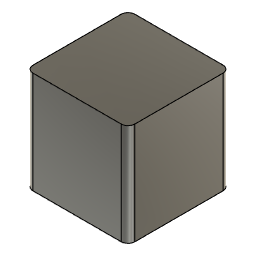
Head v1 (Autodesk Fusion 360 design; units mm, degrees)
Autodesk Fusion 360 part; units mm, degrees
sketch "Sketch1" plane through (0, 0, 0) normal (0, 0, 1) x (1, 0, 0)
  line L0 (15, -15) -> (-15, -15)
  line L1 (-15, -15) -> (-15, 15)
  line L2 (-15, 15) -> (15, 15)
  line L3 (15, 15) -> (15, -15)
  line L4 (15, -15) -> (-15, 15) construction
  line L5 (-15, -15) -> (15, 15) construction
  dimension "d1" = 30
  dimension "d2" = 30
  constraint horizontal L0
  constraint perpendicular L0 L1
  constraint parallel L0 L2
  constraint parallel L1 L3
  constraint coincident L4 origin
  constraint coincident L5 origin
  measures "d1" distance of L1.end L2.end
  measures "d2" distance of L0.end L1.end
extrude "Extrude1" add sketch "Sketch1" along normal blind 30
fillet "Fillet1" radius 2 4 edges at (-15, -15, 15) (15, -15, 15) (15, 15, 15) (-15, 15, 15)
shell "Shell1" thickness 1.6 removed faces 1 at (4.3333, -5, 30)
sketch "Sketch2" plane through (0, 0, 30) normal (0, 0, 1) x (-1, 0, 0)
  arc A0 (-13.4, -13) -> (-13, -13.4) centre (-13, -13) ccw
  line L0 (-13.4, -13) -> (-13.4, 13)
  arc A1 (-13, 13.4) -> (-13.4, 13) centre (-13, 13) ccw
  line L1 (-13, 13.4) -> (13, 13.4)
  arc A2 (13.4, 13) -> (13, 13.4) centre (13, 13) ccw
  line L2 (13.4, 13) -> (13.4, -13)
  arc A3 (13, -13.4) -> (13.4, -13) centre (13, -13) ccw
  line L3 (13, -13.4) -> (-13, -13.4)
  arc A4 (13, -15) -> (15, -13) centre (13, -13) ccw
  line L4 (15, -13) -> (15, 13)
  arc A5 (15, 13) -> (13, 15) centre (13, 13) ccw
  line L5 (13, 15) -> (-13, 15)
  arc A6 (-13, 15) -> (-15, 13) centre (-13, 13) ccw
  line L6 (-15, 13) -> (-15, -13)
  arc A7 (-15, -13) -> (-13, -15) centre (-13, -13) ccw
  line L7 (-13, -15) -> (13, -15)
extrude "Extrude2" add sketch "Sketch2" against normal blind 1.6 contours A0 L0 A1 L1 A2 L2 A3 L3
